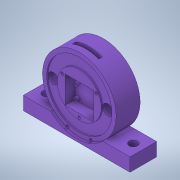
# Autodesk Inventor part: MountForLightRingAndPiCamera
Saved by Autodesk Inventor 2020.1 (Build 241239000, 239)
## iProperties
Created: 2018-12-23
Part Number: MountForLightRingAndPiCamera
Material: PBT Plastic
Document SubType Name: Modeling
Designer: steele
Density: 1.31 g/cm^3
Appearance: Violet
LightRingExternalDiameter: 2.362 in
LightRingInternalDiameter: 1.732 in
LightRingDepth: 0.047 in
LightRingSpacing: 0.079 in
MountExternalDiameter: 2.756 in
CameraCenterToTop: 0.373 in
CameraCenterToBottom: 0.567 in
CameraCenterToSide: 0.492 in
CameraLensToSurface: 0.197 in
CameraBoardThickness: 0.039 in
CameraRibbonHolderThickness: 0.134 in
LightRingWireDiameter: 0.315 in
CameraHoleDiameter: 0.087 in
CameraSpacing: 0.039 in
MountDepth: 0.500 in
CameraRibbonHolderWidth: 0.984 in
DepthForCamera: 0.370 in
CoverDepth: 0.100 in
LightRingCenterRadius: 1.024 in
LightRingCenterDiameter: 2.047 in
LightRingLightWidth: 0.079 in
LightRingLightLength: 0.157 in
SupportScrewsDiameter: 1.477 in
Number8ScrewDiameter: 0.177 in
ScrewOffset: 30.00 deg
Author: steele
Autodesk Inventor part; units mm, degrees
ref_plane "YZ Plane" through (0, 0, 0) normal (1, 0, 0) x (0, 1, 0)
ref_plane "XZ Plane" through (0, 0, 0) normal (0, 1, 0) x (-1, 0, 0)
ref_plane "XY Plane" through (0, 0, 0) normal (0, 0, 1) x (1, 0, 0)
sketch "Sketch1" plane through (0, 0, 0) normal (0, 0, 1) x (1, 0, 0)
  circle A0 centre (0, 0) radius 35
  dimension "d0" = 70
  constraints: 1 centre point, 1 coincident
  measures "d0" diameter of A0
extrude "Extrusion1" add sketch "Sketch1" against normal blind 22.86
sketch "Sketch2" plane through (0, 0, 0) normal (0, 0, 1) x (1, 0, 0)
  circle A0 centre (0, 0) radius 31
  circle A1 centre (0, 0) radius 21
  dimension "d3" = 62
  dimension "d4" = 42
  constraints: 2 centre point, 2 coincident
  measures "d3" diameter of A0
  measures "d4" diameter of A1
extrude "Extrusion2" cut sketch "Sketch2" against normal blind 1.2
sketch "Sketch7" plane through (0, 0, 0) normal (0, 0, 1) x (1, 0, 0)
  line L0 (-13.5, -15.4) -> (13.5, -15.4)
  line L1 (13.5, -15.4) -> (13.5, 10.462)
  line L2 (13.5, 10.462) -> (-13.5, 10.462)
  line L3 (-13.5, 10.462) -> (-13.5, -15.4)
  point P0 (0, 0)
  dimension "d24" = 10.462
  dimension "d25" = 15.4
  dimension "d27" = 13.5
  dimension "d28" = 13.5
  constraints: 8 end point, 2 parallel, 1 horizontal, 1 perpendicular
  measures "d24" distance from line of L2 point (0, 0)
  measures "d25" distance from line of point (0, 0) L0
  measures "d27" distance from line of point (0, 0) L3
  measures "d28" distance from line of point (0, 0) L1
extrude "Extrusion4" cut sketch "Sketch7" against normal blind 9.4
sketch "Sketch10" plane through (-13.5, 10.462, 0) normal (0, -1, 0) x (1, 0, 0)
  line L0 (-21.5, -22.86) -> (48.5, -22.86) construction
  line L1 (13.5, -9.4) -> (26, -9.4)
  line L2 (26, -9.4) -> (26, -6)
  line L3 (26, -6) -> (13.5, -6)
  line L4 (13.5, -6) -> (13.5, -9.4)
  line L5 (34.5, 0) -> (-7.5, 0) projected
  line L6 (13.5, -9.4) -> (1, -9.4)
  line L7 (1, -9.4) -> (1, -6)
  line L8 (1, -6) -> (13.5, -6)
  line L9 (13.5, 0) -> (13.5, -6) construction
  line L10 (13.5, -9.4) -> (13.5, -22.86) construction
  dimension "d33" = 9.4
  dimension "d34" = 12.5
  dimension "d35" = 3.4
  constraints: 18 end point, 2 parallel, 1 horizontal, 1 midpoint, 1 perpendicular
  measures "d33" distance between parallel lines of L1 L5
  measures "d34" distance of L2.end L3.end
  measures "d35" distance of L1.end L2.end
extrude "Extrusion5" cut sketch "Sketch10" against normal through all
sketch "Sketch20" plane through (0, 0, 0) normal (0, 0, 1) x (1, 0, 0)
  arc A0 (0, -35) -> (24.9337, -24.5624) centre (0, 0) ccw
  line L0 (0, -24.5624) -> (24.9337, -24.5624) construction
  circle A1 centre (0, 0) radius 35 construction
  line L1 (24.9337, -24.5624) -> (50.8, -24.5624)
  line L2 (50.8, -24.5624) -> (50.8, -37.2624)
  line L3 (50.8, -37.2624) -> (0, -37.2624)
  line L4 (0, -35) -> (0, -37.2624)
  arc A2 (-24.9337, -24.5624) -> (0, -35) centre (0, 0) ccw
  line L5 (-24.9337, -24.5624) -> (-50.8, -24.5624)
  line L6 (-50.8, -24.5624) -> (-50.8, -37.2624)
  line L7 (-50.8, -37.2624) -> (0, -37.2624)
  dimension "d76" = 10.4376
  dimension "d77" = 50.8
  dimension "d78" = 12.7
  constraints: 19 end point, 6 point on circle, 3 symmetric about line, 2 centre point, 2 horizontal, 2 perpendicular, 1 coincident, 1 vertical, 1 other
  measures "d76" distance edge to line of A0 L0
  measures "d77" distance of L2.end L3.end
  measures "d78" distance of L1.end L2.end
extrude "Extrusion11" add sketch "Sketch20" against normal blind 22.86
sketch "Sketch24" plane through (0, 0, -1.2) normal (0, 0, 1) x (1, 0, 0)
  circle A0 centre (-26, 0) radius 5
  circle A1 centre (0, 0) radius 26 construction
  circle A2 centre (26, 0) radius 5
  dimension "d95" = 26
  dimension "d96" = 10
  dimension "d99" = 360
  constraints: 2 centre point, 1 coincident, 1 horizontal alignment, 7 other
  measures "d95" distance of A0.centre point (0, 0)
  measures "d96" diameter of A0
extrude "Extrusion14" cut sketch "Sketch24" against normal through all
sketch "Sketch27" plane through (0, 0, 0) normal (0, 0, 1) x (1, 0, 0)
  line L0 (50.8, -37.2624) -> (-50.8, -37.2624) projected
  line L1 (-50.8, -24.5624) -> (50.8, -24.5624) projected
  line L2 (-50.8, -37.2624) -> (50.8, -37.2624)
  line L3 (50.8, -37.2624) -> (50.8, -24.5624)
  line L4 (-50.8, -24.5624) -> (-50.8, -37.2624)
  arc A0 (-24.6756, -24.5624) -> (24.6756, -24.5624) centre (0, 0) ccw
  line L5 (50.8, -24.5624) -> (24.6756, -24.5624)
  line L6 (-24.6756, -24.5624) -> (-50.8, -24.5624)
  constraints: 10 end point, 3 parallel, 2 point on circle, 1 centre point, 1 coincident, 1 horizontal, 1 perpendicular
extrude "Extrusion16" add sketch "Sketch27" along normal blind 2.54 contours L0 L4 L1 A0 L3
sketch "Sketch43" plane through (-50.8, -37.2624, -22.86) normal (0, -1, 0) x (1, 0, 0)
  line L0 (0, 25.4) -> (0, 0) construction
  line L1 (0, 12.7) -> (101.6, 12.7) construction
  line L2 (101.6, 0) -> (101.6, 25.4) construction
  point P0 (50.8, 22.86)
  point P1 (9.525, 12.7)
  point P2 (92.075, 12.7)
  point P3 (68.2625, 49.2125)
  dimension "d192" = 9.525
  dimension "d193" = 9.525
  constraints: 2 end point, 2 midpoint, 2 point on line
  measures "d192" distance from line of point (9.525, 12.7) L0
  measures "d193" distance from line of point (92.075, 12.7) L2
hole "Hole for 1/4 0.266 diam" at (-41.275, -37.2624, -10.16) at (41.275, -37.2624, -10.16) at (17.4625, -37.2624, 26.3525) direction (0, 1, 0) diameter 6.7564 end through all clearance for "Flat Head Machine Screw (82)" size "1/4" standard "Ansi Unified Screw Threads"
sketch "Sketch44" plane through (24.9337, -24.5624, -22.86) normal (0, 1, 0) x (1, 0, 0)
  circle A0 centre (16.3413, -12.7) radius 3.3782 projected
  circle A1 centre (-66.2087, -12.7) radius 3.3782 projected
  point P0 (-24.9337, -22.86)
  constraints: 2 coincident
hole "Hole for 1/4 Insert" at (41.275, -24.5624, -10.16) at (-41.275, -24.5624, -10.16) direction (0, -1, 0) diameter 8.0264 depth 7.9248
sketch "Sketch16" plane through (0, 0, -9.4) normal (0, 0, 1) x (1, 0, 0)
  circle A0 centre (-10.5, 0) radius 2.0828
  circle A1 centre (10.5, 0) radius 2.0828
  circle A2 centre (-10.5, -12.58) radius 2.0828
  circle A3 centre (10.5, -12.58) radius 2.0828
  point P0 (0, 0)
  dimension "d66" = 4.1656
  constraints: 4 centre point, 3 equal radius
  measures "d66" diameter of A0
extrude "Extrusion To Support Camera" add sketch "Sketch16" along normal blind 2.7
sketch "Sketch45" plane through (-10.5, -12.58, -6.7) normal (0, 0, 1) x (1, 0, 0)
  circle A0 centre (0, 0) radius 2.0828 projected
  circle A1 centre (0, 12.58) radius 2.0828 projected
  circle A2 centre (21, 12.58) radius 2.0828 projected
  circle A3 centre (21, 0) radius 2.0828 projected
  point P0 (10.5, 12.58)
  constraints: 4 coincident
hole "Hole for 2-56 threads for camera" at (-10.5, -12.58, -6.7) at (-10.5, 0, -6.7) at (10.5, 0, -6.7) at (10.5, -12.58, -6.7) direction (0, 0, -1) diameter 1.7018 end through all
sketch "Sketch46" plane through (0, 0, -22.86) normal (0, 0, -1) x (-1, 0, 0)
  circle A0 centre (10.5, 0) radius 0.8509 projected
  circle A1 centre (10.5, -12.58) radius 0.8509 projected
  circle A2 centre (-10.5, -12.58) radius 0.8509 projected
  circle A3 centre (-10.5, 0) radius 0.8509 projected
  point P0 (0, 0)
  constraints: 4 coincident
hole "Hole for 2-56 insert" at (-10.5, 0, -22.86) at (-10.5, -12.58, -22.86) at (10.5, -12.58, -22.86) at (10.5, 0, -22.86) direction (0, 0, 1) diameter 3.2639 depth 3.9878
sketch "Sketch36" plane through (0, 0, -22.86) normal (0, 0, -1) x (-1, 0, 0)
  point P0 (0, 0)
  point P1 (-11.123, -31.7252)
  point P2 (11.102, -31.7252)
hole "Hole for 6-32 threads for battery holder" at (11.123, -31.7252, -22.86) at (-11.102, -31.7252, -22.86) direction (0, 0, 1) diameter 2.6416 end through all counterbore diameter 4.8514 counterbore depth 7.1374 thread size "6-32 UNC" class "2B" standard "ANSI Unified Screw Threads"
sketch "Sketch51" plane through (0, 0, -22.86) normal (0, 0, -1) x (-1, 0, 0)
  circle A0 centre (0, 0) radius 18.7521 construction
  point P0 (0, -18.7521)
  point P1 (16.2398, 9.376)
  point P2 (-16.2398, 9.3761)
  dimension "d262" = 37.5042
  dimension "d265" = 360
  constraints: 1 coincident, 1 vertical alignment, 6 other
hole "Hole20" at (0, -18.7521, -22.86) at (-16.2398, 9.376, -22.86) at (16.2398, 9.3761, -22.86) direction (0, 0, 1) diameter 2.6416 end through all counterbore diameter 4.8514 counterbore depth 7.1374 thread size "6-32 UNC" class "2B" standard "ANSI Unified Screw Threads"
equation "\"d0\" = MountExternalDiameter"
equation "\"d3\" = LightRingExternalDiameter + LightRingSpacing"
equation "\"d4\" = LightRingInternalDiameter - LightRingSpacing"
equation "\"d5\" = LightRingDepth"
equation "\"d24\" = CameraCenterToTop + CameraSpacing"
equation "\"d25\" = CameraCenterToBottom + CameraSpacing"
equation "\"d27\" = CameraCenterToSide + CameraSpacing"
equation "\"d28\" = CameraCenterToSide + CameraSpacing"
equation "\"d31\" = DepthForCamera"
equation "\"d33\" = DepthForCamera"
equation "\"d34\" = 0.5 * CameraRibbonHolderWidth"
equation "\"d35\" = CameraRibbonHolderThickness"
equation "\"d95\" = LightRingCenterRadius"
equation "\"d262\" = SupportScrewsDiameter"
equation "\"LightRingExternalDiameter\" = 60"
equation "\"LightRingInternalDiameter\" = 44"
equation "\"LightRingDepth\" = 1.2"
equation "\"LightRingSpacing\" = 2"
equation "\"LightRingCenterRadius\" = 0.5 * LightRingCenterDiameter"
equation "\"CameraCenterToTop\" = 9.462"
equation "\"CameraCenterToBottom\" = 14.4"
equation "\"CameraCenterToSide\" = 12.5"
equation "\"CameraLensToSurface\" = 5"
equation "\"CameraBoardThickness\" = 1"
equation "\"CameraRibbonHolderThickness\" = 3.4"
equation "\"LightRingWireDiameter\" = 8"
equation "\"CameraHoleDiameter\" = 2.2"
equation "\"CameraSpacing\" = 1"
equation "\"MountDepth\" = 12.7"
equation "\"CameraRibbonHolderWidth\" = 25"
equation "\"DepthForCamera\" = CameraBoardThickness + CameraLensToSurface + CameraRibbonHolderThickness"
equation "\"CoverDepth\" = 2.54"
equation "\"LightRingCenterDiameter\" = 52"
equation "\"LightRingLightLength\" = 4"
equation "\"LightRingLightWidth\" = 2"
equation "\"Number8ScrewDiameter\" = 4.4958"
equation "\"ScrewOffset\" = 30deg"
equation "\"MountExternalDiameter\" = 70"
equation "\"SupportScrewsDiameter\" = 37.5042"
body "Solid1"
